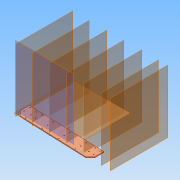
# Autodesk Inventor part: Pancake_Timing Backboard 2_4 Lanes
Saved by Autodesk Inventor 2018.1 (Build 221171000, 171)
## iProperties
Created: 2019-02-22
Part Number: Pancake_Timing Backboard 2_4 Lanes
Material: Wood (Oak)
Document SubType Name: Modeling
Designer: James
Density: 0.76 g/cm^3
Appearance: White Oak - Natural Medium Gloss
Mass: 79.783 g
Surface Area: 478.752 cm^2
Volume: 104.978 cm^3
Author: James
Autodesk Inventor part; units mm, degrees
ref_plane "YZ Plane" through (0, 0, 0) normal (1, 0, 0) x (0, 1, 0)
ref_plane "XZ Plane" through (0, 0, 0) normal (0, 1, 0) x (-1, 0, 0)
ref_plane "XY Plane" through (0, 0, 0) normal (0, 0, 1) x (1, 0, 0)
derived "Pancake_Skeleton.ipt"
ref_plane "Ground" through (0, 0, 0) normal (0, 1, 0) x (-1, 0, 0)
ref_plane "Back" through (0, 0, 0) normal (0, 0, 1) x (1, 0, 0)
ref_plane "LHS" through (0, 0, 0) normal (1, 0, 0) x (0, 1, 0)
ref_plane "Lane 1" through (90, 0, 0) normal (1, 0, 0) x (0, 1, 0)
ref_plane "Lane 2" through (185, 0, 0) normal (1, 0, 0) x (0, 1, 0)
ref_plane "Lane 3" through (280, 0, 0) normal (1, 0, 0) x (0, 1, 0)
ref_plane "Lane 4" through (375, 0, 0) normal (1, 0, 0) x (0, 1, 0)
ref_plane "Lane 5" through (470, 0, 0) normal (1, 0, 0) x (0, 1, 0)
ref_plane "RHS" through (520, 0, 0) normal (1, 0, 0) x (0, 1, 0)
sketch "Sketch1" plane through (0, 0, 0) normal (0, 0, 1) x (1, 0, 0)
  line L0 (0, 79.6154) -> (0, -13.2692) projected
  line L1 (0, 16.3462) -> (425, 0)
  line L2 (425, 0) -> (425, 50)
  line L3 (425, 50) -> (0, 66.3462)
  line L4 (0, 66.3462) -> (0, 16.3462)
  line L5 (-85, 0) -> (510, 0) projected
  line L6 (520, 79.6154) -> (520, -13.2692) projected
  dimension "d31" = 50
  dimension "d61" = 2.203
  dimension "d62" = 95
  constraints: 8 end point, 2 parallel, 1 collinear, 1 point on line, 1 vertical
  measures "d31" distance of L1.end L2.end
  measures "d61" angle of L5 L1
  measures "d62" distance between parallel lines of L6 L2
extrude "Extrusion1" add sketch "Sketch1" along normal blind 5 contours L3 L2 L1 L0
sketch "Sketch2" plane through (0, 0, 5) normal (0, 0, 1) x (1, 0, 0)
  line L0 (90, 79.6154) -> (90, -13.2692) projected
  line L1 (425, 50) -> (0, 66.3462) projected
  line L2 (-104, 0) -> (624, 0) projected
  line L3 (185, 84) -> (185, -14) projected
  line L4 (0, 84) -> (0, -14) projected
  line L5 (0, 16.3462) -> (425, 0) projected
  point P0 (0, 0)
  point P1 (50, 54.4231)
  point P2 (50, 24.4231)
  dimension "d4" = 30
  dimension "d29" = 95
  dimension "d30" = 50
  dimension "d33" = 9.9926
  dimension "d34" = 9.9926
  constraints: 1 vertical alignment
  measures "d4" distance of point (50, 24.423) point (50, 54.423)
  measures "d29" distance between parallel lines of L3 L0
  measures "d30" distance from line of point (50, 54.423) L4
  measures "d33" distance from line of L1 point (50, 54.423)
  measures "d34" distance from line of L5 point (50, 24.423)
hole "Hole1" at (50, 54.4231, 5) at (50, 24.4231, 5) direction (0, 0, -1) diameter 4.5 end through all clearance for "Socket Head Cap Screw" size "M4" standard "Ansi Metric M Profile"
pattern_linear "Rectangular Pattern1" count 4 spacing 95 along (0.9992612, -0.0384331, 0) of "Hole1"
sketch "Sketch3" plane through (0, 0, 5) normal (0, 0, 1) x (1, 0, 0)
  line L0 (425, 50) -> (0, 66.3462) projected
  line L1 (-104, 0) -> (624, 0) projected
  line L2 (0, 84) -> (0, -14) projected
  line L3 (0, 16.3462) -> (425, 0) projected
  line L4 (520, 84) -> (520, -14) projected
  point P0 (0, 0)
  point P1 (12.5, 58.8462)
  point P2 (12.5, 23.8462)
  point P3 (412.5, 42.5)
  point P4 (412.5, 7.5)
  dimension "d20" = 12.5
  dimension "d36" = 35
  dimension "d38" = 107.5
  dimension "d39" = 35
  dimension "d41" = 7.5
  dimension "d42" = 7.5
  constraints: 2 vertical alignment, 1 other
  measures "d20" distance from line of L2 point (12.5, 58.846)
  measures "d36" distance of point (12.5, 23.846) point (12.5, 58.846)
  measures "d39" distance of point (412.5, 7.5) point (412.5, 42.5)
  measures "d41" vertical distance of L0.start point (412.5, 42.5)
  measures "d42" vertical distance of point (12.5, 58.846) L0.end
hole "Hole2" at (12.5, 58.8462, 5) at (12.5, 23.8462, 5) at (412.5, 42.5, 5) at (412.5, 7.5, 5) direction (0, 0, -1) diameter 4.5 end through all clearance for "Socket Head Cap Screw" size "M4" standard "Ansi Metric M Profile"
ref_plane "Work Plane10" through (212.5, 16.3462, 0) normal (-1, 0, 0) x (0, 0, 1)
sketch "Sketch4" plane through (0, 0, 5) normal (0, 0, 1) x (1, 0, 0)
  line L0 (80, 55.7637) -> (78.6548, 20.7895)
  line L1 (384.7747, 44.0416) -> (383.4295, 9.0674)
  line L2 (425, 50) -> (0, 66.3462) projected
  line L3 (0, 16.3462) -> (425, 0) projected
  line L4 (0, 84) -> (0, -14) projected
  line L5 (520, 84) -> (520, -14) projected
  point P0 (0, 0)
  dimension "d43" = 7.5
  dimension "d44" = 7.5
  dimension "d48" = 35
  dimension "d49" = 80
  dimension "d58" = 35
  dimension "d60" = 305
  constraints: 4 end point, 2 perpendicular, 1 other
  measures "d43" distance from line of L2 L0.start
  measures "d44" distance from line of L2 L1.start
  measures "d48" distance of L0.start L0.end
  measures "d49" distance from line of L0.start L4
  measures "d58" distance of L1.start L1.end
  measures "d60" distance of L1.start L0.start
hole "Hole3" at (80, 55.7637, 5) at (78.6548, 20.7895, 5) at (384.7747, 44.0416, 5) at (383.4295, 9.0674, 5) direction (0, 0, -1) diameter 4.5 end through all clearance for "Flat Head Machine Screw" size "M4" standard "Ansi Metric M Profile"
sketch "Sketch5" plane through (0, 0, 5) normal (0, 0, 1) x (1, 0, 0)
  circle A0 centre (384.7747, 44.0416) radius 2.25 projected
  circle A1 centre (80, 55.7637) radius 2.25 projected
  circle A2 centre (78.6548, 20.7895) radius 2.25 projected
  circle A3 centre (383.4295, 9.0674) radius 2.25 projected
  circle A4 centre (412.5, 42.5) radius 2.25 projected
  circle A5 centre (12.5, 58.8462) radius 2.25 projected
  circle A6 centre (12.5, 23.8462) radius 2.25 projected
  circle A7 centre (412.5, 7.5) radius 2.25 projected
  circle A8 centre (334.7894, 43.4696) radius 2.25 projected
  circle A9 centre (334.7894, 13.4696) radius 2.25 projected
  circle A10 centre (239.8596, 47.1208) radius 2.25 projected
  circle A11 centre (239.8596, 17.1208) radius 2.25 projected
  circle A12 centre (144.9298, 50.7719) radius 2.25 projected
  circle A13 centre (144.9298, 20.7719) radius 2.25 projected
  circle A14 centre (50, 54.4231) radius 2.25 projected
  circle A15 centre (50, 24.4231) radius 2.25 projected
  line L0 (0, 16.3462) -> (425, 0) projected
  line L1 (425, 0) -> (425, 50) projected
  line L2 (425, 50) -> (0, 66.3462) projected
  line L3 (0, 66.3462) -> (0, 16.3462) projected
  line L4 (0, 66.3462) -> (0, 16.3462) projected
  line L5 (0, 16.3462) -> (0, -8.6538)
  line L6 (0, -8.6538) -> (425, -25)
  line L7 (425, -25) -> (425, 0)
  line L8 (0, 16.3462) -> (425, 0) projected
  point P0 (0, 0)
  dimension "d63" = 25
  constraints: 6 end point, 2 parallel, 1 vertical
  measures "d63" distance of L6.end L0.end
extrude "Extrusion2" add sketch "Sketch5" against normal up to surface (5 mm away) contours L0 L7 L6 L5
sketch "Sketch6" plane through (0, 0, 5) normal (0, 0, 1) x (1, 0, 0)
  circle A0 centre (50, 24.4231) radius 2.25 projected
  point P0 (0, 0)
  point P1 (50, -4.5769)
  dimension "d66" = 29
  constraints: 1 vertical alignment
  measures "d66" distance of point (50, -4.577) A0.centre
hole "Hole4" at (50, -4.5769, 5) direction (0, 0, -1) diameter 4.5 end through all clearance for "Flat Head Machine Screw" size "M4" standard "Ansi Metric M Profile"
pattern_linear "Rectangular Pattern2" count 4 spacing 95 along (0.9992612, -0.0384331, 0) of "Hole4"
chamfer "Chamfer1" distance 25 angle 45 2 edges at (0, -8.6538, 2.5) (425, -25, 2.5)
equation "\"d33\" = d34"
equation "\"d44\" = d43"
equation "\"d58\" = d48"
body "Solid1"
